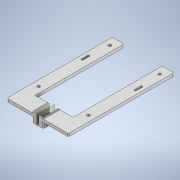
# Autodesk Inventor part: Hộp đựng động cơ
Saved by Autodesk Inventor 2020 (Build 240168000, 168)
## iProperties
Created: 2022-04-01
Part Number: Hộp đựng động cơ
Material: Generic
Document SubType Name: Modeling
Designer: PC
Density: 1 g/cm^3
Appearance: Default
Author: PC
Autodesk Inventor part; units mm, degrees
ref_plane "YZ Plane" through (0, 0, 0) normal (1, 0, 0) x (0, 1, 0)
ref_plane "XZ Plane" through (0, 0, 0) normal (0, 1, 0) x (-1, 0, 0)
ref_plane "XY Plane" through (0, 0, 0) normal (0, 0, 1) x (1, 0, 0)
sketch "Sketch1" plane through (0, 0, 0) normal (0, 1, 0) x (-1, 0, 0)
  line L0 (0, 0) -> (-27, 0)
  line L1 (-27, 0) -> (-27, -39)
  line L2 (-27, -39) -> (0, -39)
  line L3 (0, -39) -> (0, 0)
  dimension "d0" = 27
  dimension "d1" = 39
  constraints: 8 end point, 2 parallel, 1 horizontal, 1 perpendicular
  measures "d0" distance of L2.end L1.end
  measures "d1" distance of L0.end L1.end
extrude "Extrusion1" add sketch "Sketch1" along normal blind 22
sketch "Sketch2" plane through (0, 22, 0) normal (0, 1, 0) x (1, 0, 0)
  line L0 (27, 39) -> (0, 39) projected
  line L1 (2, 39) -> (2, 2)
  line L2 (2, 2) -> (25, 2)
  line L3 (25, 2) -> (25, 39)
  line L4 (27, 0) -> (27, 39) projected
  line L5 (0, 39) -> (0, 0) projected
  line L6 (0, 0) -> (27, 0) projected
  dimension "d4" = 2
  dimension "d5" = 2
  dimension "d6" = 2
  constraints: 6 end point, 2 perpendicular, 2 point on line, 1 vertical
  measures "d4" distance between parallel lines of L4 L3
  measures "d5" distance between parallel lines of L1 L5
  measures "d6" distance between parallel lines of L6 L2
extrude "Extrusion2" cut sketch "Sketch2" against normal blind 20 contours L3 L2 L1 L0
sketch "Sketch3" plane through (0, 2, 0) normal (0, 1, 0) x (1, 0, 0)
  circle A0 centre (13.5, 13.2) radius 2.75
  line L0 (25, 2) -> (2, 2) projected
  circle A1 centre (22, 34) radius 1.5
  circle A2 centre (5, 34) radius 1.5
  line L1 (2, 39) -> (25, 39) projected
  line L2 (27, 0) -> (27, 39) projected
  line L3 (0, 39) -> (0, 0) projected
  point P0 (20, 2)
  point P1 (7, 2)
  point P2 (27, 5)
  point P3 (0, 5)
  dimension "d10" = 5.5
  dimension "d11" = 11.2
  dimension "d20" = 3
  dimension "d21" = 3
  dimension "d23" = 0
  dimension "d24" = 5
  dimension "d25" = 5
  dimension "d59" = 32
  constraints: 3 centre point
  measures "d10" diameter of A0
  measures "d11" distance from line of L0 A0.centre
  measures "d20" diameter of A1
  measures "d21" diameter of A2
  measures "d23" vertical distance of A2.centre A1.centre
  measures "d24" distance from line of L2 A1.centre
  measures "d25" distance from line of L3 A2.centre
  measures "d59" distance from line of L0 A2.centre
extrude "Extrusion3" cut sketch "Sketch3" against normal through all
sketch "Sketch5" plane through (0, 22, 0) normal (0, 1, 0) x (1, 0, 0)
  line L0 (0, 0) -> (27, 0) projected
  line L1 (13.5, 0) -> (13.5, 2)
  line L2 (25, 2) -> (2, 2) projected
  line L3 (10.8, 0) -> (16.2, 0)
  line L4 (16.2, 0) -> (16.2, 2)
  line L5 (16.2, 2) -> (10.8, 2)
  line L6 (10.8, 2) -> (10.8, 0)
  line L7 (10.8, 0) -> (16.2, 2) construction
  line L8 (16.2, 0) -> (10.8, 2) construction
  point P0 (5, 0)
  point P1 (22, 0)
  point P2 (20, 2)
  point P3 (7, 2)
  point P4 (13.5, 1)
  dimension "d17" = 5.4
  constraints: 14 end point, 5 midpoint, 2 parallel, 1 horizontal, 1 perpendicular, 1 point on line
  measures "d17" distance of L5.end L4.end
extrude "Extrusion4" cut sketch "Sketch5" against normal through all
sketch "Sketch6" plane through (27, 0, 0) normal (1, 0, 0) x (0, 0, -1)
  line L0 (0, 22) -> (0, 0) projected
  line L1 (39, 2) -> (39, 22) projected
  line L2 (0, 20) -> (39, 20)
  line L3 (39, 20) -> (39, 13)
  line L4 (39, 13) -> (0, 13)
  line L5 (0, 13) -> (0, 20)
  point P0 (0, 13)
  dimension "d26" = 7
  constraints: 8 end point, 2 parallel, 2 point on line, 1 horizontal, 1 perpendicular
  measures "d26" distance of L2.end L3.end
extrude "Extrusion5" add sketch "Sketch6" along normal blind 60
ref_plane "Work Plane1" through (13.5, 22, -39) normal (-1, 0, 0) x (0, 0, 1)
sketch "Sketch7" plane through (27, 0, -39) normal (0, 0, -1) x (-1, 0, 0)
  line L0 (-60, 13) -> (-60, 20) projected
  line L1 (0, 13) -> (-60, 13) projected
  line L2 (-60, 20) -> (-32, 20)
  line L3 (-32, 20) -> (-32, 13)
  line L4 (-32, 13) -> (-60, 13)
  line L5 (-60, 13) -> (-60, 20)
  point P0 (27, 0)
  dimension "d29" = 28
  constraints: 8 end point, 2 parallel, 1 horizontal, 1 perpendicular, 1 point on line
  measures "d29" distance of L3.end L4.end
extrude "Extrusion6" add sketch "Sketch7" along normal blind 213
sketch "Sketch8" plane through (27, 20, 0) normal (0, 1, 0) x (1, 0, 0)
  circle A0 centre (46, 61.8594) radius 3.25
  line L0 (60, 0) -> (60, 252) projected
  circle A1 centre (46, 231.9406) radius 3.25
  point P0 (-27, 0)
  dimension "d32" = 6.5
  dimension "d33" = 14
  dimension "d34" = 6.5
  dimension "d35" = 14
  constraints: 2 centre point
  measures "d32" diameter of A0
  measures "d33" distance from line of L0 A0.centre
  measures "d34" diameter of A1
  measures "d35" distance from line of L0 A1.centre
hole "Hole1" at (73, 20, -61.8594) at (73, 20, -231.9406) direction (0, -1, 0) diameter 4 end through all counterbore diameter 6.5 counterbore depth 4
sketch "Sketch9" plane through (27, 13, -39) normal (0, -1, 0) x (1, 0, 0)
  arc A0 (54.25, -131) -> (45.75, -131) centre (50, -131) ccw
  line L0 (60, 39) -> (60, -213) projected
  line L1 (0, 39) -> (60, 39) projected
  arc A1 (45.75, -146) -> (54.25, -146) centre (50, -146) ccw
  line L2 (54.25, -131) -> (54.25, -146)
  line L3 (45.75, -146) -> (45.75, -131)
  point P0 (-27, 39)
  dimension "d43" = 8.5
  dimension "d44" = 10
  dimension "d45" = 170
  dimension "d46" = 8.5
  dimension "d47" = 15
  constraints: 4 end point, 4 point on circle, 2 centre point, 2 tangent
  measures "d43" diameter of A0
  measures "d44" distance from line of L0 A0.centre
  measures "d45" distance from line of L1 A0.centre
  measures "d46" diameter of A1
  measures "d47" distance of A1.centre A0.centre
extrude "Extrusion7" cut sketch "Sketch9" against normal blind 4
sketch "Sketch10" plane through (27, 17, -39) normal (0, -1, 0) x (1, 0, 0)
  arc A0 (52.25, -131) -> (47.75, -131) centre (50, -131) ccw
  line L0 (60, 39) -> (60, -213) projected
  line L1 (0, 39) -> (60, 39) projected
  arc A1 (47.75, -146) -> (52.25, -146) centre (50, -146) ccw
  line L2 (47.75, -146) -> (47.75, -131)
  line L3 (52.25, -131) -> (52.25, -146)
  point P0 (-27, 39)
  dimension "d50" = 4.5
  dimension "d51" = 10
  dimension "d52" = 170
  dimension "d53" = 4.5
  dimension "d54" = 15
  constraints: 5 point on circle, 4 end point, 2 centre point, 1 parallel, 1 vertical
  measures "d50" diameter of A0
  measures "d51" distance from line of L0 A0.centre
  measures "d52" distance from line of L1 A0.centre
  measures "d53" diameter of A1
  measures "d54" distance of A1.centre A0.centre
extrude "Extrusion8" cut sketch "Sketch10" against normal blind 4
mirror "Mirror2" about plane through (13.5, 22, -39) normal (-1, 0, 0) of "Extrusion5"
mirror "Mirror3" about plane through (13.5, 22, -39) normal (-1, 0, 0) of "Extrusion6", "Hole1", "Extrusion8", "Extrusion7"
fillet "Fillet2" radius 3 10 edges at (87, 16.5, -252) (59, 16.5, -252) (-32, 16.5, -252) (-60, 16.5, -252) (-60, 16.5, 0) (87, 16.5, 0) (27, 6.5, 0) (27, 21, 0) (0, 6.5, 0) (0, 21, 0)
fillet "Fillet3" radius 2 2 edges at (26, 22, -39) (1, 22, -39)
body "Solid1"
